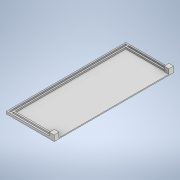
# Autodesk Inventor part: Bottom
Saved by Autodesk Inventor 2022 (Build 260153000, 153)
## iProperties
Created: 2021-07-04
Part Number: Bottom
Material: Generic
Document SubType Name: Modeling
Designer: Matthijs
Density: 1 g/cm^3
Appearance: Default
Author: Matthijs
Autodesk Inventor part; units mm, degrees
ref_plane "YZ Plane" through (0, 0, 0) normal (1, 0, 0) x (0, 1, 0)
ref_plane "XZ Plane" through (0, 0, 0) normal (0, 1, 0) x (-1, 0, 0)
ref_plane "XY Plane" through (0, 0, 0) normal (0, 0, 1) x (1, 0, 0)
sketch "Sketch2" plane through (0, 0, 0) normal (0, 1, 0) x (-1, 0, 0)
  line L0 (-50, -125) -> (50, -125)
  line L1 (50, -125) -> (50, 125)
  line L2 (50, 125) -> (-50, 125)
  line L3 (-50, 125) -> (-50, -125)
  line L4 (-50, -125) -> (50, 125) construction
  line L5 (50, -125) -> (-50, 125) construction
  point P0 (0, 0)
  dimension "d4" = 250
  dimension "d5" = 100
  constraints: 12 end point, 2 midpoint, 2 parallel, 1 horizontal, 1 perpendicular
  measures "d4" distance of L0.end L1.end
  measures "d5" distance of L1.end L2.end
extrude "Extrusion2" add sketch "Sketch2" along normal blind 2
sketch "Sketch6" plane through (0, 2, 0) normal (0, 1, 0) x (1, 0, 0)
  line L0 (-50, 125) -> (-50, -125) projected
  line L1 (50, 125) -> (-50, 125) projected
  line L2 (-50, -125) -> (-47, -125)
  line L3 (-47, -125) -> (-47, 125)
  line L4 (-47, 125) -> (-50, 125)
  line L5 (-50, 125) -> (-50, -125)
  point P0 (0, 0)
  dimension "d11" = 3
  constraints: 8 end point, 2 parallel, 1 horizontal, 1 perpendicular, 1 point on line
  measures "d11" distance of L4.end L3.end
extrude "Extrusion4" add sketch "Sketch6" along normal blind 3
sketch "Sketch7" plane through (0, 2, 0) normal (0, 1, 0) x (1, 0, 0)
  line L0 (-50, -125) -> (50, -125) projected
  line L1 (50, 125) -> (-50, 125) projected
  line L2 (-44, -125) -> (-41, -125)
  line L3 (-41, -125) -> (-41, 125)
  line L4 (-41, 125) -> (-44, 125)
  line L5 (-44, 125) -> (-44, -125)
  line L6 (-47, 125) -> (-47, -125) projected
  point P0 (0, 0)
  dimension "d14" = 3
  dimension "d15" = 3
  constraints: 8 end point, 2 parallel, 2 point on line, 1 horizontal, 1 perpendicular
  measures "d14" distance of L4.end L3.end
  measures "d15" distance between parallel lines of L6 L5
extrude "Extrusion5" add sketch "Sketch7" along normal blind 3 contours L5 L1 L3 L0
sketch "Sketch8" plane through (0, 2, 0) normal (0, 1, 0) x (1, 0, 0)
  line L0 (50, -125) -> (50, 125) projected
  line L1 (-50, -125) -> (50, -125)
  line L2 (50, -125) -> (50, -122)
  line L3 (50, -122) -> (-50, -122)
  line L4 (-50, -122) -> (-50, -125)
  point P0 (0, 0)
  dimension "d18" = 3
  constraints: 8 end point, 2 parallel, 1 horizontal, 1 perpendicular, 1 point on line
  measures "d18" distance of L2.end L1.end
extrude "Extrusion6" add sketch "Sketch8" along normal blind 3
sketch "Sketch9" plane through (0, 2, 0) normal (0, 1, 0) x (1, 0, 0)
  line L0 (50, 125) -> (-50, 125) projected
  line L1 (50, -125) -> (50, 125) projected
  line L2 (-50, 125) -> (50, 125)
  line L3 (50, 125) -> (50, 122)
  line L4 (50, 122) -> (-50, 122)
  line L5 (-50, 122) -> (-50, 125)
  point P0 (0, 0)
  dimension "d21" = 3
  constraints: 8 end point, 2 parallel, 1 horizontal, 1 perpendicular, 1 point on line
  measures "d21" distance of L2.end L3.end
extrude "Extrusion7" add sketch "Sketch9" along normal blind 3
sketch "Sketch10" plane through (0, 2, 0) normal (0, 1, 0) x (1, 0, 0)
  line L0 (-50, -125) -> (50, -125) projected
  line L1 (50, -125) -> (40, -125)
  line L2 (40, -125) -> (40, -115)
  line L3 (40, -115) -> (50, -115)
  line L4 (50, -115) -> (50, -125)
  point P0 (0, 0)
  dimension "d24" = 10
  dimension "d25" = 10
  constraints: 8 end point, 2 parallel, 1 horizontal, 1 perpendicular
  measures "d24" distance of L2.end L3.end
  measures "d25" distance of L1.end L2.end
extrude "Extrusion8" add sketch "Sketch10" along normal blind 10
sketch "Sketch11" plane through (0, 2, 0) normal (0, 1, 0) x (1, 0, 0)
  line L0 (50, 125) -> (40, 125)
  line L1 (40, 125) -> (40, 115)
  line L2 (40, 115) -> (50, 115)
  line L3 (50, 115) -> (50, 125)
  point P0 (0, 0)
  dimension "d28" = 10
  dimension "d29" = 10
  constraints: 8 end point, 2 parallel, 1 horizontal, 1 perpendicular
  measures "d28" distance of L1.end L2.end
  measures "d29" distance of L0.end L1.end
extrude "Extrusion9" add sketch "Sketch11" along normal blind 10
sketch "Sketch12" plane through (0, 2, 0) normal (0, 1, 0) x (1, 0, 0)
  line L0 (-41, -122) -> (-41, 122) projected
  line L1 (50, -125) -> (50, 125) projected
  line L2 (-41, -119) -> (50, -119)
  line L3 (50, -119) -> (50, -116)
  line L4 (50, -116) -> (-41, -116)
  line L5 (-41, -116) -> (-41, -119)
  line L6 (40, -122) -> (-41, -122) projected
  point P0 (0, 0)
  point P1 (-41, -116)
  dimension "d32" = 3
  dimension "d33" = 3
  constraints: 8 end point, 2 parallel, 2 point on line, 1 horizontal, 1 perpendicular
  measures "d32" distance of L3.end L2.end
  measures "d33" distance between parallel lines of L6 L2
extrude "Extrusion10" add sketch "Sketch12" along normal blind 3
sketch "Sketch13" plane through (0, 2, 0) normal (0, 1, 0) x (1, 0, 0)
  line L0 (-41, 122) -> (-41, -116) projected
  line L1 (50, -115) -> (50, 115) projected
  line L2 (-41, 119) -> (50, 119)
  line L3 (50, 119) -> (50, 116)
  line L4 (50, 116) -> (-41, 116)
  line L5 (-41, 116) -> (-41, 119)
  line L6 (-41, 122) -> (40, 122) projected
  point P0 (0, 0)
  dimension "d36" = 3
  dimension "d37" = 3
  constraints: 8 end point, 2 parallel, 2 point on line, 1 horizontal, 1 perpendicular
  measures "d36" distance of L2.end L3.end
  measures "d37" distance between parallel lines of L6 L2
extrude "Extrusion11" add sketch "Sketch13" along normal blind 3
body "Solid2"
